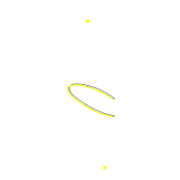
# Autodesk Inventor part: Radius_cover_strip
Saved by Autodesk Inventor 2022 (Build 260153000, 153)
## iProperties
Created: 2022-07-25
Part Number: Radius_cover_strip
Material: Generic
Document SubType Name: Modeling
Designer: dell
Density: 1 g/cm^3
Appearance: Default
Author: dell
Autodesk Inventor part; units mm, degrees
ref_plane "YZ Plane" through (0, 0, 0) normal (1, 0, 0) x (0, 1, 0)
ref_plane "XZ Plane" through (0, 0, 0) normal (0, 1, 0) x (-1, 0, 0)
ref_plane "XY Plane" through (0, 0, 0) normal (0, 0, 1) x (1, 0, 0)
sketch "Sketch3" plane through (0, 0, 0) normal (0, 0, 1) x (1, 0, 0)
  spline S0 degree 5 poles (0, 0) (-0.3974, 2.0072) (0.1969, 5.498) (4.1668, 10.4426) (6.6937, 12.3831) (11.9329, 16.3087) (16.249, 18.7393) (21.0357, 21.2745) (25.6905, 23.4082) (30.4194, 25.4123) (35.1553, 27.2371) (39.924, 28.9391) (44.7108, 30.5191) (49.5184, 31.995) (54.3424, 33.3733) (59.1821, 34.6624) (64.0352, 35.868) (68.9007, 36.9951) (73.7771, 38.0478) (78.6634, 39.03) (83.5586, 39.9446) (88.4617, 40.7944) (93.3719, 41.5819) (98.2885, 42.3091) (103.2107, 42.9782) (108.1378, 43.5908) (113.0694, 44.1485) (118.0047, 44.6527) (122.9434, 45.105) (127.8848, 45.5064) (132.8285, 45.8581) (137.7741, 46.1613) (142.7212, 46.4168) (147.6693, 46.6257) (152.6182, 46.7888) (157.5673, 46.9071) (162.5168, 46.981) (167.4649, 47.0118) (172.4151, 46.9994) (177.3557, 46.9459) (182.3067, 46.8492) (187.2158, 46.7162) (192.1973, 46.5336) (196.995, 46.3322) (201.9013, 46.1019) (206.7513, 45.8489) (211.6198, 45.571) (216.4766, 45.2698) (221.3369, 44.9451) (226.194, 44.5975) (231.0504, 44.2274) (235.905, 43.835) (240.7581, 43.4209) (245.6095, 42.9852) (250.4593, 42.5283) (255.3072, 42.0505) (260.1533, 41.5521) (264.9975, 41.0333) (269.8397, 40.4944) (274.68, 39.9357) (279.5182, 39.3573) (284.3542, 38.7595) (289.1882, 38.1424) (294.0199, 37.5063) (298.8494, 36.8513) (303.6765, 36.1777) (308.5014, 35.4854) (313.3238, 34.7748) (318.1438, 34.0459) (322.9614, 33.2988) (327.7764, 32.5337) (332.5889, 31.7506) (337.3988, 30.9496) (342.206, 30.1309) (347.0106, 29.2944) (351.8124, 28.4403) (356.6115, 27.5685) (361.4077, 26.6792) (366.2011, 25.7723) (370.9916, 24.8479) (375.7791, 23.906) (380.5637, 22.9466) (385.3452, 21.9696) (390.1237, 20.9751) (394.899, 19.9631) (399.6711, 18.9334) (404.44, 17.8861) (409.2057, 16.8211) (413.9679, 15.7384) (418.7271, 14.6378) (423.4818, 13.5194) (428.2357, 12.3827) (432.9796, 11.2288) (437.7349, 10.0547) (442.4515, 8.8669) (447.2458, 7.6499) (451.8472, 6.4396) (456.8839, 5.1519) (460.896, 3.9819) (467.2752, 2.476) (468.1448, 1.687) (481.7015, -0.8179) (467.9699, 0.3048) (466.921, -0.2606) (460.3834, -0.0983) (456.2125, -0.2527) (451.0297, -0.2748) (446.2874, -0.3579) (441.3612, -0.419) (436.5195, -0.494) (431.6468, -0.5677) (426.7926, -0.6467) (421.9355, -0.7284) (417.0848, -0.8141) (412.2362, -0.9032) (407.3916, -0.9961) (402.5501, -1.0929) (397.712, -1.1935) (392.8771, -1.298) (388.0453, -1.4065) (383.2167, -1.519) (378.3912, -1.6355) (373.5687, -1.7561) (368.7492, -1.8807) (363.9326, -2.0094) (359.119, -2.1421) (354.3082, -2.2788) (349.5002, -2.4195) (344.695, -2.5641) (339.8925, -2.7127) (335.0927, -2.8651) (330.2955, -3.0213) (325.501, -3.1811) (320.709, -3.3446) (315.9195, -3.5116) (311.1325, -3.682) (306.3479, -3.8557) (301.5657, -4.0325) (296.7859, -4.2124) (292.0083, -4.3951) (287.233, -4.5805) (282.4599, -4.7684) (277.6889, -4.9587) (272.9201, -5.151) (268.1533, -5.3454) (263.3885, -5.5414) (258.6257, -5.7388) (253.8648, -5.9375) (249.1057, -6.1371) (244.3484, -6.3374) (239.5927, -6.538) (234.8388, -6.7387) (230.0864, -6.9391) (225.3357, -7.1389) (220.5858, -7.3377) (215.839, -7.5351) (211.0888, -7.7309) (206.3503, -7.9242) (201.5931, -8.1154) (196.8927, -8.3019) (192.0833, -8.488) (187.4565, -8.6638) (182.7593, -8.8567) (178.1025, -9.0532) (173.436, -9.2584) (168.7788, -9.4692) (164.1195, -9.6862) (159.4617, -9.9081) (154.8033, -10.1344) (150.1448, -10.3643) (145.4854, -10.597) (140.825, -10.8315) (136.1631, -11.067) (131.4993, -11.3024) (126.8331, -11.5367) (122.1641, -11.7686) (117.4918, -11.9971) (112.8156, -12.2206) (108.1349, -12.4378) (103.4492, -12.6471) (98.7577, -12.8466) (94.0597, -13.0345) (89.3545, -13.2086) (84.6411, -13.3665) (79.9186, -13.5053) (75.1859, -13.6221) (70.4418, -13.7131) (65.6849, -13.7743) (60.9134, -13.8005) (56.126, -13.7861) (51.319, -13.7232) (46.4925, -13.6043) (41.636, -13.4143) (36.7599, -13.1465) (31.8194, -12.7603) (26.8873, -12.2726) (21.679, -11.516) (16.9108, -10.7238) (10.741, -8.9628) (7.7374, -8.0433) (2.2608, -4.9859) (0.3958, -1.9991) (0, 0) knots 0 0 0 0 0 0 0.007489 0.012112 0.017774 0.023064 0.028281 0.033461 0.038617 0.043757 0.048885 0.054005 0.059118 0.064225 0.069327 0.074426 0.079521 0.084614 0.089704 0.094792 0.099878 0.104963 0.110046 0.115127 0.120208 0.125287 0.130366 0.135443 0.14052 0.145596 0.150671 0.155746 0.16082 0.165893 0.170967 0.176039 0.181111 0.186183 0.191255 0.196326 0.201386 0.206438 0.211482 0.216518 0.221546 0.226577 0.231609 0.23664 0.241672 0.246704 0.251736 0.256768 0.2618 0.266832 0.271865 0.276897 0.28193 0.286963 0.291996 0.297029 0.302062 0.307095 0.312128 0.317162 0.322196 0.32723 0.332264 0.337298 0.342332 0.347367 0.352401 0.357436 0.362471 0.367506 0.372542 0.377577 0.382613 0.387649 0.392685 0.397722 0.402758 0.407795 0.412833 0.41787 0.422908 0.427946 0.432985 0.438023 0.443063 0.448102 0.453142 0.458182 0.463223 0.468264 0.473306 0.478348 0.483391 0.488434 0.493477 0.498521 0.503565 0.508608 0.51365 0.518689 0.523727 0.528763 0.533797 0.538828 0.543858 0.548886 0.553912 0.558937 0.563959 0.56898 0.573999 0.579017 0.584032 0.589046 0.594059 0.59907 0.604079 0.609087 0.614093 0.619098 0.624102 0.629104 0.634104 0.639104 0.644101 0.649098 0.654093 0.659087 0.66408 0.669071 0.674061 0.67905 0.684038 0.689025 0.69401 0.698995 0.703978 0.70896 0.713941 0.718922 0.723901 0.728879 0.733856 0.738832 0.743808 0.748782 0.753756 0.758728 0.7637 0.768671 0.773642 0.778612 0.783581 0.788552 0.793515 0.798469 0.803415 0.808351 0.813276 0.8182 0.823124 0.828048 0.832972 0.837896 0.84282 0.847745 0.85267 0.857597 0.862524 0.867452 0.872382 0.877313 0.882247 0.887182 0.89212 0.897061 0.902005 0.906953 0.911904 0.91686 0.921821 0.926788 0.931761 0.936742 0.941731 0.94673 0.95174 0.956765 0.961808 0.966873 0.971969 0.977111 0.982337 0.987951 0.992541 1 1 1 1 1 1
  point P0 (7.5036, 12.949)
  point P1 (11.9443, 16.1143)
  point P2 (16.4858, 18.8224)
  point P3 (21.0951, 21.2234)
  point P4 (25.755, 23.3946)
  point P5 (30.4548, 25.3817)
  point P6 (35.1872, 27.2149)
  point P7 (39.9471, 28.9151)
  point P8 (44.7305, 30.4976)
  point P9 (49.5343, 31.9741)
  point P10 (54.3561, 33.3536)
  point P11 (59.1936, 34.6436)
  point P12 (64.0452, 35.85)
  point P13 (68.9094, 36.9778)
  point P14 (73.7848, 38.0313)
  point P15 (78.6702, 39.014)
  point P16 (83.5646, 39.9291)
  point P17 (88.467, 40.7794)
  point P18 (93.3767, 41.5673)
  point P19 (98.2928, 42.295)
  point P20 (103.2145, 42.9644)
  point P21 (108.1413, 43.5773)
  point P22 (113.0725, 44.1353)
  point P23 (118.0075, 44.6399)
  point P24 (122.9459, 45.0924)
  point P25 (127.887, 45.4941)
  point P26 (132.8305, 45.8461)
  point P27 (137.7759, 46.1494)
  point P28 (142.7227, 46.4052)
  point P29 (147.6707, 46.6143)
  point P30 (152.6193, 46.7776)
  point P31 (157.5683, 46.896)
  point P32 (162.5174, 46.9702)
  point P33 (167.4661, 47.001)
  point P34 (172.4142, 46.9891)
  point P35 (177.3614, 46.9351)
  point P36 (182.3075, 46.8397)
  point P37 (187.2521, 46.7035)
  point P38 (192.1951, 46.527)
  point P39 (197.0288, 46.3247)
  point P40 (201.8925, 46.096)
  point P41 (206.7551, 45.8427)
  point P42 (211.6166, 45.5652)
  point P43 (216.4769, 45.264)
  point P44 (221.3359, 44.9394)
  point P45 (226.1935, 44.5919)
  point P46 (231.0497, 44.2218)
  point P47 (235.9044, 43.8296)
  point P48 (240.7574, 43.4155)
  point P49 (245.6089, 42.9799)
  point P50 (250.4586, 42.5231)
  point P51 (255.3065, 42.0454)
  point P52 (260.1525, 41.547)
  point P53 (264.9967, 41.0283)
  point P54 (269.839, 40.4895)
  point P55 (274.6792, 39.9308)
  point P56 (279.5174, 39.3525)
  point P57 (284.3534, 38.7547)
  point P58 (289.1873, 38.1377)
  point P59 (294.019, 37.5016)
  point P60 (298.8485, 36.8467)
  point P61 (303.6756, 36.1731)
  point P62 (308.5005, 35.4809)
  point P63 (313.3229, 34.7703)
  point P64 (318.1429, 34.0414)
  point P65 (322.9604, 33.2943)
  point P66 (327.7754, 32.5292)
  point P67 (332.5879, 31.7462)
  point P68 (337.3977, 30.9452)
  point P69 (342.2049, 30.1265)
  point P70 (347.0095, 29.2901)
  point P71 (351.8113, 28.4359)
  point P72 (356.6103, 27.5642)
  point P73 (361.4065, 26.6749)
  point P74 (366.1999, 25.768)
  point P75 (370.9903, 24.8437)
  point P76 (375.7779, 23.9017)
  point P77 (380.5624, 22.9423)
  point P78 (385.3439, 21.9654)
  point P79 (390.1223, 20.9709)
  point P80 (394.8976, 19.9588)
  point P81 (399.6697, 18.9292)
  point P82 (404.4385, 17.8819)
  point P83 (409.2041, 16.8169)
  point P84 (413.9664, 15.7341)
  point P85 (418.7253, 14.6335)
  point P86 (423.4807, 13.515)
  point P87 (428.2326, 12.3786)
  point P88 (432.981, 11.224)
  point P89 (437.7257, 10.0513)
  point P90 (442.4667, 8.8603)
  point P91 (447.2041, 7.6508)
  point P92 (451.9375, 6.4229)
  point P93 (456.6671, 5.1762)
  point P94 (461.3928, 3.9108)
  point P95 (466.1144, 2.6264)
  point P96 (470.8319, 1.3228)
  point P97 (475.5453, 0)
  point P98 (470.6516, -0.0527)
  point P99 (465.7622, -0.1076)
  point P100 (460.8768, -0.165)
  point P101 (455.9955, -0.225)
  point P102 (451.1181, -0.2878)
  point P103 (446.2446, -0.3534)
  point P104 (441.3749, -0.4221)
  point P105 (436.509, -0.4939)
  point P106 (431.6468, -0.569)
  point P107 (426.7882, -0.6475)
  point P108 (421.9331, -0.7295)
  point P109 (417.0816, -0.815)
  point P110 (412.2335, -0.9042)
  point P111 (407.3887, -0.9972)
  point P112 (402.5474, -1.0939)
  point P113 (397.7092, -1.1945)
  point P114 (392.8744, -1.2991)
  point P115 (388.0427, -1.4076)
  point P116 (383.2141, -1.5201)
  point P117 (378.3886, -1.6366)
  point P118 (373.5662, -1.7572)
  point P119 (368.7467, -1.8818)
  point P120 (363.9302, -2.0105)
  point P121 (359.1166, -2.1432)
  point P122 (354.3058, -2.2799)
  point P123 (349.4979, -2.4206)
  point P124 (344.6927, -2.5652)
  point P125 (339.8903, -2.7137)
  point P126 (335.0905, -2.8661)
  point P127 (330.2934, -3.0223)
  point P128 (325.4989, -3.1821)
  point P129 (320.7069, -3.3456)
  point P130 (315.9175, -3.5126)
  point P131 (311.1305, -3.6829)
  point P132 (306.3459, -3.8566)
  point P133 (301.5638, -4.0334)
  point P134 (296.784, -4.2132)
  point P135 (292.0064, -4.3958)
  point P136 (287.2312, -4.5812)
  point P137 (282.4581, -4.7691)
  point P138 (277.6872, -4.9593)
  point P139 (272.9184, -5.1516)
  point P140 (268.1516, -5.3459)
  point P141 (263.3869, -5.5418)
  point P142 (258.6241, -5.7392)
  point P143 (253.8632, -5.9378)
  point P144 (249.1041, -6.1373)
  point P145 (244.3469, -6.3375)
  point P146 (239.5913, -6.5381)
  point P147 (234.8374, -6.7387)
  point P148 (230.0851, -6.939)
  point P149 (225.3343, -7.1387)
  point P150 (220.5849, -7.3374)
  point P151 (215.8369, -7.5348)
  point P152 (211.0903, -7.7303)
  point P153 (206.3448, -7.9237)
  point P154 (201.6005, -8.1145)
  point P155 (196.8572, -8.3022)
  point P156 (192.0839, -8.4873)
  point P157 (187.4199, -8.6686)
  point P158 (182.7576, -8.8582)
  point P159 (178.0967, -9.0555)
  point P160 (173.4369, -9.2599)
  point P161 (168.778, -9.4707)
  point P162 (164.1198, -9.6874)
  point P163 (159.4618, -9.9092)
  point P164 (154.8039, -10.1353)
  point P165 (150.1455, -10.365)
  point P166 (145.4865, -10.5974)
  point P167 (140.8264, -10.8317)
  point P168 (136.1648, -11.0669)
  point P169 (131.5013, -11.302)
  point P170 (126.8355, -11.5359)
  point P171 (122.1669, -11.7676)
  point P172 (117.4949, -11.9956)
  point P173 (112.8191, -12.2188)
  point P174 (108.1389, -12.4356)
  point P175 (103.4537, -12.6444)
  point P176 (98.7628, -12.8434)
  point P177 (94.0655, -13.0308)
  point P178 (89.361, -13.2042)
  point P179 (84.6484, -13.3614)
  point P180 (79.9268, -13.4995)
  point P181 (75.1952, -13.6154)
  point P182 (70.4524, -13.7055)
  point P183 (65.6971, -13.7654)
  point P184 (60.9276, -13.7904)
  point P185 (56.1424, -13.7742)
  point P186 (51.3393, -13.7097)
  point P187 (46.5157, -13.5876)
  point P188 (41.6686, -13.3964)
  point P189 (36.7941, -13.1207)
  point P190 (31.8869, -12.7396)
  point P191 (26.9398, -12.223)
  point P192 (21.9421, -11.525)
  point P193 (16.8766, -10.5685)
  point P194 (11.7103, -9.2033)
  point P195 (6.3612, -7.0418)
  constraints: 1 coincident, 198 other
extrude "Extrusion1" add sketch "Sketch3" along normal blind 4
shell "Shell1" thickness 3 outward yes removed faces 2 at (233.006, 10.3252, 4) at (233.006, 10.3252, 0)
thicken "Thicken1" operation add thickness 2 both sides no extend neighbours yes toward (-0.0367814, 0.9993233, 0) faces at (305.2513, -6.8988, 1.3333)
sketch "Sketch37" plane through (0, 0, 4) normal (0, 0, 1) x (1, 0, 0)
  line L0 (0, 32.0227) -> (0, -17.6611)
  line L1 (0, -17.6611) -> (10, -17.6611)
  line L2 (10, -17.6611) -> (10, 32.0227)
  line L3 (10, 32.0227) -> (0, 32.0227)
  line L4 (0, 77.6157) -> (0, -68.7441)
  line L5 (0, -68.7441) -> (120, -68.7441)
  line L6 (120, -68.7441) -> (120, 77.6157)
  line L7 (120, 77.6157) -> (0, 77.6157)
  line L8 (0, 180.4775) -> (0, -167.7743)
  line L9 (0, -167.7743) -> (575.1059, -167.7743)
  line L10 (575.1059, -167.7743) -> (575.1059, 180.4775)
  line L11 (575.1059, 180.4775) -> (0, 180.4775)
  line L12 (0, 58.0292) -> (0, -41.7314)
  line L13 (0, -41.7314) -> (-48.6852, -41.7314)
  line L14 (-48.6852, -41.7314) -> (-48.6852, 58.0292)
  line L15 (-48.6852, 58.0292) -> (0, 58.0292)
  point P0 (0, 0)
  point P1 (0, -17.6611)
  dimension "d161" = 10
  dimension "d162" = 120
  constraints: 32 end point, 8 parallel, 4 perpendicular, 3 point on line, 3 vertical
  measures "d161" distance between parallel lines of L0 L2
  measures "d162" distance of L4.end L5.end
extrude "Extrusion16" cut sketch "Sketch37" against normal blind 10 contours L8 L11 L10 L9 L5 L6 L7
ref_plane "Work Plane4" through (0, 0, 2) normal (0, 0, 1) x (1, 0, 0)
sketch "Sketch40" plane through (0, 0, 4) normal (0, 0, 1) x (1, 0, 0)
  spline S0 degree 5 poles (120, 45.833) (113.0104, 45.1869) (106.0326, 44.4123) (99.0705, 43.5026) (92.129, 42.4487) (82.701, 40.7976) (80.191, 40.3367) (77.6849, 39.8544) (75.1832, 39.3499) (69.419, 38.1324) (66.1583, 37.4026) (62.9049, 36.6311) (59.6601, 35.8152) (54.3319, 34.3928) (52.2427, 33.8141) (50.158, 33.2143) (48.0783, 32.5924) (43.7363, 31.2414) (41.477, 30.5084) (39.2274, 29.7459) (36.989, 28.9518) (33.4579, 27.6388) (32.1572, 27.142) (30.8615, 26.6321) (29.5714, 26.1085) (26.2514, 24.72) (24.2304, 23.8342) (22.2218, 22.9193) (20.2438, 21.94) (17.2917, 20.4011) (16.3288, 19.8852) (15.37, 19.3586) (14.4038, 18.8096) (12.4669, 17.6481) (11.4952, 17.037) (10.5249, 16.3868) (9.5626, 15.7155) (7.4502, 14.1844) (6.3521, 13.3493) (5.3047, 12.5123) (4.2185, 11.5437) (1.4928, 8.4814) (0.1434, 6.6359) (-0.9357, 4.4844) (-1.4573, 2.0931) (-0.981, -0.1942) knots 0 0 0 0 0 0 0.264715 0.264715 0.264715 0.264715 0.360952 0.360952 0.360952 0.360952 0.486888 0.486888 0.486888 0.486888 0.568378 0.568378 0.568378 0.568378 0.657467 0.657467 0.657467 0.657467 0.709692 0.709692 0.709692 0.709692 0.792448 0.792448 0.792448 0.792448 0.834556 0.834556 0.834556 0.834556 0.876664 0.876664 0.876664 0.876664 0.930032 0.930032 0.930032 0.930032 1 1 1 1 1 1 projected
  spline S1 degree 5 poles (0, 0) (-0.423, 2.0385) (0.0607, 4.1609) (1.0242, 6.0763) (2.1967, 7.7241) (4.8656, 10.8047) (6.0351, 11.836) (7.1932, 12.7408) (8.4616, 13.698) (10.763, 15.3323) (11.7126, 15.9814) (12.6647, 16.5984) (13.6178, 17.1817) (15.5254, 18.2971) (16.4801, 18.829) (17.4348, 19.3455) (18.3982, 19.8551) (21.1755, 21.2821) (22.9715, 22.1598) (24.7785, 22.9787) (26.5863, 23.7723) (29.6925, 25.0775) (30.9745, 25.6004) (32.2622, 26.1096) (33.5548, 26.6056) (37.0666, 27.9173) (39.294, 28.7108) (41.5324, 29.4726) (43.7807, 30.205) (48.1027, 31.5551) (50.1737, 32.1769) (52.2501, 32.7766) (54.3313, 33.3553) (59.6399, 34.778) (62.8734, 35.5941) (66.116, 36.3661) (69.3665, 37.0964) (75.1137, 38.3151) (77.6082, 38.8202) (80.1071, 39.3031) (82.6101, 39.7645) (92.0499, 41.4246) (99.0109, 42.4854) (105.9927, 43.4005) (112.9904, 44.1794) (120, 44.8287) knots 0 0 0 0 0 0 0.062895 0.062895 0.062895 0.062895 0.123114 0.123114 0.123114 0.123114 0.164977 0.164977 0.164977 0.164977 0.206839 0.206839 0.206839 0.206839 0.282294 0.282294 0.282294 0.282294 0.334919 0.334919 0.334919 0.334919 0.424792 0.424792 0.424792 0.424792 0.507038 0.507038 0.507038 0.507038 0.634144 0.634144 0.634144 0.634144 0.731289 0.731289 0.731289 0.731289 1 1 1 1 1 1 projected
  spline S2 degree 5 poles (120, -11.8739) (108.1413, -12.4533) (96.2807, -12.9993) (84.4173, -13.4575) (72.5451, -13.7824) (57.0151, -13.7931) (53.358, -13.7654) (49.7011, -13.7017) (46.0452, -13.5935) (40.4526, -13.3428) (38.5141, -13.2404) (36.5768, -13.1188) (34.6409, -12.9758) (31.5379, -12.7114) (30.3694, -12.604) (29.2021, -12.4866) (28.0362, -12.3572) (25.7928, -12.0825) (24.7151, -11.9407) (23.6434, -11.7875) (22.5761, -11.6285) (20.4419, -11.2829) (19.3748, -11.0975) (18.3037, -10.89) (17.2185, -10.6547) (15.0947, -10.1491) (14.087, -9.8862) (13.1129, -9.6209) (12.1758, -9.3528) (10.324, -8.7689) (9.4091, -8.4532) (8.48, -8.0919) (7.4807, -7.6446) (4.7904, -6.1838) (3.0424, -5.0691) (1.4543, -3.6205) (0.3537, -1.876) (0, 0) knots 0 0 0 0 0 0 0.492436 0.492436 0.492436 0.492436 0.644117 0.644117 0.644117 0.644117 0.724629 0.724629 0.724629 0.724629 0.773276 0.773276 0.773276 0.773276 0.818322 0.818322 0.818322 0.818322 0.863369 0.863369 0.863369 0.863369 0.904089 0.904089 0.904089 0.904089 0.944809 0.944809 0.944809 0.944809 1 1 1 1 1 1 projected
  spline S3 degree 5 poles (-0.981, -0.1942) (-0.5836, -2.3054) (0.6289, -4.189) (2.2295, -5.6992) (3.9911, -6.883) (7.0497, -8.5481) (8.0935, -9.0155) (9.0596, -9.3908) (10.0022, -9.7159) (11.8957, -10.313) (12.8467, -10.5849) (13.8296, -10.8525) (14.8462, -11.1179) (17.0027, -11.6313) (18.1052, -11.8703) (19.192, -12.0808) (20.2718, -12.2684) (22.4263, -12.6173) (23.5012, -12.7774) (24.5785, -12.9313) (25.6617, -13.0739) (27.9222, -13.3507) (29.0954, -13.4809) (30.27, -13.5991) (31.4457, -13.7072) (34.564, -13.9728) (36.5079, -14.1164) (38.4533, -14.2386) (40.3998, -14.3414) (46.0095, -14.5929) (49.6745, -14.7015) (53.3405, -14.7654) (57.0067, -14.7931) (72.5456, -14.7824) (84.4177, -14.4581) (96.2809, -14.0001) (108.1414, -13.4544) (120, -12.8751) knots 0 0 0 0 0 0 0.063557 0.063557 0.063557 0.063557 0.10431 0.10431 0.10431 0.10431 0.145063 0.145063 0.145063 0.145063 0.189974 0.189974 0.189974 0.189974 0.234886 0.234886 0.234886 0.234886 0.283258 0.283258 0.283258 0.283258 0.363146 0.363146 0.363146 0.363146 0.513403 0.513403 0.513403 0.513403 1 1 1 1 1 1 projected
  arc A0 (120, 37.8287) -> (51.5312, 32.5573) centre (98.5463, -130.8121) ccw
  arc A1 (120, 38.8287) -> (50.6394, 33.3405) centre (98.6066, -131.8356) ccw
  line L0 (120, 38.8287) -> (120, 37.8287)
  line L1 (120, 44.8287) -> (120, 45.833) projected
  arc A2 (46.0271, -13.5716) -> (120, -1.8739) centre (52.6451, 184.3177) ccw
  arc A3 (45.1185, -14.5407) -> (120, -2.8739) centre (52.3277, 185.3294) ccw
  line L2 (120, -2.8739) -> (120, -1.8739)
  line L3 (120, -12.8751) -> (120, -11.8739) projected
  line L4 (120, -12.8751) -> (120, -11.8739) projected
  line L5 (120, 44.8287) -> (120, 45.833) projected
  line L6 (120, 44.8287) -> (120, 45.833) projected
  line L7 (120, -12.8751) -> (120, -11.8739) projected
  point P0 (38.5007, -13.2281)
  point P1 (72.2656, -13.6744)
  point P2 (78.5542, 38.9915)
  point P3 (78.2087, -13.5444)
  point P4 (36.3467, -15.0951)
  point P5 (78.5542, 38.9915)
  dimension "d167" = 1
  dimension "d168" = 170
  dimension "d169" = 172
  dimension "d171" = 1
  dimension "d183" = 9
  dimension "d185" = 6
  dimension "d186" = 198
  dimension "d187" = 200
  constraints: 8 point on circle, 4 centre point, 4 end point, 2 collinear, 2 vertical, 19 other
  measures "d167" distance of L0.start L0.end
  measures "d168" radius of A0
  measures "d169" radius of A1
  measures "d171" distance of L2.start L2.end
  measures "d183" distance of L3.end L2.start
  measures "d185" distance of L1.start L0.start
  measures "d186" radius of A2
  measures "d187" radius of A3
extrude "Extrusion18" add sketch "Sketch40" against normal blind 4 contours A1 L0 A0 S1 | S2 A2 L2 A3
extrude "Extrusion19" cut sketch "Sketch40" against normal blind 10 contours L1 S1 A1 S0 | A3 S2 L3 S3
sketch "Sketch42" plane through (0, 0, 4) normal (0, 0, 1) x (1, 0, 0)
  arc A0 (120, 37.8287) -> (51.5312, 32.5573) centre (98.5463, -130.8121) ccw projected
  arc A1 (46.0271, -13.5716) -> (120, -1.8739) centre (52.6451, 184.3177) ccw projected
  line L0 (120, -1.8739) -> (120, -2.8739) projected
  arc A2 (45.1185, -14.5407) -> (120, -2.8739) centre (52.3277, 185.3294) ccw projected
  arc A3 (120, 38.8287) -> (50.6394, 33.3405) centre (98.6066, -131.8356) ccw projected
  line L1 (120, 38.8287) -> (120, 37.8287) projected
  constraints: 4 other
sketch "Sketch39" plane through (0, 0, 0) normal (0, 0, -1) x (-1, 0, 0)
  line L0 (26.854, 76.2259) -> (-213.6331, 76.2259)
  line L1 (-213.6331, 76.2259) -> (-213.6331, 3.9927)
  line L2 (-213.6331, 3.9927) -> (26.854, 3.9927)
  line L3 (26.854, 3.9927) -> (26.854, 76.2259)
  line L4 (60.7949, 3.9927) -> (-257.1471, 3.9927)
  line L5 (-257.1471, 3.9927) -> (-257.1471, -75.4928)
  line L6 (-257.1471, -75.4928) -> (60.7949, -75.4928)
  line L7 (60.7949, -75.4928) -> (60.7949, 3.9927)
  point P0 (0, 0)
  point P1 (26.854, 3.9927)
  point P2 (-213.6331, 3.9927)
  constraints: 16 end point, 4 parallel, 2 horizontal, 2 perpendicular, 1 point on line
body "Solid1"
